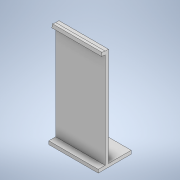
# Autodesk Inventor part: Holder
Saved by Autodesk Inventor 2021 (Build 250183000, 183)
## iProperties
Created: 2020-06-26
Part Number: Holder
Material: Generic
Document SubType Name: Modeling
Designer: Mariano
Density: 1 g/cm^3
Appearance: Default
Author: Mariano
Autodesk Inventor part; units mm, degrees
ref_plane "YZ Plane" through (0, 0, 0) normal (1, 0, 0) x (0, 1, 0)
ref_plane "XZ Plane" through (0, 0, 0) normal (0, 1, 0) x (-1, 0, 0)
sketch "Sketch1" plane through (0, 0, 0) normal (0, 1, 0) x (-1, 0, 0)
  line L0 (15, -10) -> (-15, -10)
  line L1 (-15, -10) -> (-15, 10)
  line L2 (-15, 10) -> (15, 10)
  line L3 (15, 10) -> (15, -10)
  line L4 (15, -10) -> (-15, 10) construction
  line L5 (-15, -10) -> (15, 10) construction
  point P0 (0, 0)
  dimension "d0" = 30
  dimension "d1" = 20
  constraints: 12 end point, 2 midpoint, 2 parallel, 1 horizontal, 1 perpendicular
  measures "d0" distance of L1.end L2.end
  measures "d1" distance of L0.end L1.end
extrude "Extrusion1" add sketch "Sketch1" along normal blind 2
sketch "Sketch3" plane through (0, 0, 0) normal (0, -1, 0) x (1, 0, 0)
  line L0 (-15, 5.7967) -> (15, 5.7967)
  line L1 (15, 5.7967) -> (15, 3.7967)
  line L2 (15, 3.7967) -> (-15, 3.7967)
  line L3 (-15, 3.7967) -> (-15, 5.7967)
  line L4 (-15, 5.7967) -> (15, 3.7967) construction
  line L5 (15, 5.7967) -> (-15, 3.7967) construction
  line L6 (15, 10) -> (15, -10) projected
  point P0 (0, 4.7967)
  point P1 (15, 4.7967)
  dimension "d5" = 2
  constraints: 12 end point, 3 midpoint, 2 parallel, 1 horizontal, 1 perpendicular, 1 point on line
  measures "d5" distance between parallel lines of L2 L0
extrude "Extrusion2" add sketch "Sketch3" against normal blind 62
ref_plane "Work Plane9" through (-15, 62, 5.7967) normal (0, 0.1736482, 0.9848078) x (1, 0, 0)
sketch "Sketch10" plane through (-15, 62, 5.7967) normal (0, 0.1736482, 0.9848078) x (1, 0, 0)
  line L0 (0, -59.0885) -> (0, 0) projected
  line L1 (30, -59.0885) -> (30, 0) projected
  line L2 (0, 0) -> (30, 0)
  line L3 (30, 0) -> (30, -2)
  line L4 (30, -2) -> (0, -2)
  line L5 (0, -2) -> (0, 0)
  point P0 (15, -60.0515)
  dimension "d26" = 2
  constraints: 8 end point, 2 parallel, 1 horizontal, 1 perpendicular, 1 point on line
  measures "d26" distance between parallel lines of L2 L4
extrude "Extrusion6" add sketch "Sketch10" along normal blind 2
sketch "Sketch11" plane through (-15, 62, 5.7967) normal (0, 0.1736482, 0.9848078) x (1, 0, 0)
  line L0 (30, -2) -> (30, 0) projected
  line L1 (0, -2) -> (30, -2) projected
  line L2 (30, 0) -> (0, 0)
  line L3 (0, 0) -> (0, -2)
  line L4 (0, -2) -> (30, -2)
  line L5 (30, -2) -> (30, 0)
  point P0 (15, -60.0515)
  constraints: 8 end point, 2 parallel, 1 horizontal, 1 perpendicular
extrude "Extrusion7" add sketch "Sketch11" against normal up to surface surface through (-15, 0, 5.7967) normal (0, 0, 1)
body "Solid1"
